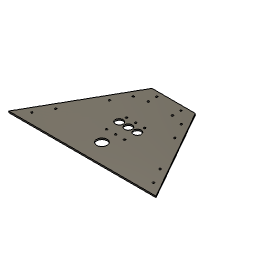
Back (Autodesk Fusion 360 design; units mm, degrees)
Autodesk Fusion 360 part; units mm, degrees
sketch "Sketch1" plane through (0, 0, 0) normal (0, 1, 0) x (1, 0, 0)
  line L0 (0, 0) -> (310.515, 0)
  line L1 (155.2575, 192.4304) -> (109.5375, 192.4304)
  line L2 (155.2575, 192.4304) -> (200.9775, 192.4304)
  line L3 (200.9775, 192.4304) -> (310.515, 0)
  line L4 (109.5375, 192.4304) -> (0, 0)
  circle A0 centre (155.2575, 96.8375) radius 8.128
  circle A1 centre (174.3075, 70.1675) radius 1.9812
  circle A2 centre (174.3075, 112.3315) radius 1.9812
  circle A3 centre (155.2575, 41.275) radius 11.1125
  circle A4 centre (136.2075, 96.8375) radius 8.128
  circle A5 centre (155.2575, 70.1675) radius 1.9812
  circle A6 centre (136.2075, 70.1675) radius 1.9812
  circle A7 centre (174.3075, 96.8375) radius 8.128
  circle A8 centre (136.2075, 112.3315) radius 1.9812
  circle A9 centre (155.2575, 112.3315) radius 1.9812
  circle A10 centre (27.0579, 21.862) radius 1.905
  circle A11 centre (86.334, 125.9954) radius 1.905
  circle A12 centre (45.2777, 53.8696) radius 1.905
  circle A13 centre (129.8575, 164.4904) radius 1.905
  circle A14 centre (129.8575, 182.2704) radius 1.905
  circle A15 centre (104.5538, 158.0031) radius 1.905
  circle A16 centre (224.181, 125.9954) radius 1.905
  circle A17 centre (265.2373, 53.8696) radius 1.905
  circle A18 centre (180.6575, 182.2704) radius 1.905
  circle A19 centre (283.4571, 21.862) radius 1.905
  circle A20 centre (180.6575, 164.4904) radius 1.905
  circle A21 centre (205.9612, 158.0031) radius 1.905
  point P0 (104.5538, 158.0031)
  point P1 (205.9612, 158.0031)
  dimension "d1" = 310.515
  dimension "d3" = 45.72
  dimension "d4" = 45.72
  dimension "d45" = 22.225
  dimension "d46" = 16.256
  dimension "d47" = 26.67
  dimension "d48" = 3.9624
  dimension "d49" = 42.164
  dimension "d50" = 3.9624
  dimension "d51" = 16.256
  dimension "d52" = 26.67
  dimension "d53" = 3.9624
  dimension "d54" = 42.164
  dimension "d55" = 3.9624
  dimension "d56" = 16.256
  dimension "d57" = 26.67
  dimension "d58" = 3.9624
  dimension "d59" = 42.164
  dimension "d60" = 3.9624
  constraint coincident L0.start L4.end
  constraint horizontal L0
  measures "d1" distance of L0.start L0.end
  measures "d3" distance of L1.start L1.end
  measures "d4" distance of L1.start L2.end
  measures "d45" diameter of A3
  measures "d46" diameter of A0
  measures "d47" distance of A5.centre A0.centre
  measures "d48" diameter of A5
  measures "d49" distance of A9.centre A5.centre
  measures "d50" diameter of A9
  measures "d51" diameter of A4
  measures "d52" distance of A4.centre A6.centre
  measures "d53" diameter of A6
  measures "d54" distance of A8.centre A6.centre
  measures "d55" diameter of A8
  measures "d56" diameter of A7
  measures "d57" distance of A1.centre A7.centre
  measures "d58" diameter of A1
  measures "d59" distance of A1.centre A2.centre
  measures "d60" diameter of A2
extrude "Extrude5" add sketch "Sketch1" along normal blind 2.794
extrude "Extrude4" [suppressed]
equation "d3 = ( 3.6 / 2 ) * 1 in"
equation "d4 = ( 3.6 / 2 ) * 1 in"
